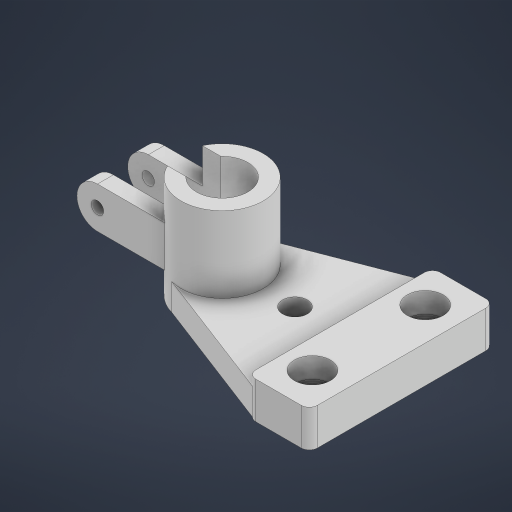
# Autodesk Inventor part: Part6
Saved by Autodesk Inventor 2023 (Build 270158000, 158)
## iProperties
Created: 2023-04-27
Part Number: Part6
Material: Ogólny
Document SubType Name: Modeling
Designer: Adam
Density: 1 g/cm^3
Appearance: Domyślna
Author: Adam
Autodesk Inventor part; units mm, degrees
ref_plane "YZ Plane" through (0, 0, 0) normal (1, 0, 0) x (0, 1, 0)
ref_plane "XZ Plane" through (0, 0, 0) normal (0, 1, 0) x (-1, 0, 0)
ref_plane "XY Plane" through (0, 0, 0) normal (0, 0, 1) x (1, 0, 0)
sketch "Szkic1" plane through (0, 0, 0) normal (0, 1, 0) x (-1, 0, 0)
  line L0 (-8, -90) -> (-52, -90)
  line L1 (-60, -82) -> (-60, 82)
  line L2 (-52, 90) -> (-8, 90)
  line L3 (0, 82) -> (0, -82)
  arc A0 (-8, -90) -> (0, -82) centre (-8, -82) ccw
  arc A1 (-60, -82) -> (-52, -90) centre (-52, -82) ccw
  arc A2 (0, 82) -> (-8, 90) centre (-8, 82) ccw
  arc A3 (-52, 90) -> (-60, 82) centre (-52, 82) ccw
  line L4 (-2.3431, -87.6569) -> (125.3697, -38.6325)
  line L5 (-2.3431, -87.6569) -> (134.4558, -87.6569) construction
  line L6 (-2.3431, 87.6569) -> (125.3697, 38.6325)
  line L7 (-2.3431, 87.6569) -> (134.4558, 87.6569) construction
  line L8 (193.533, -17) -> (224, -17)
  line L9 (224, 17) -> (193.533, 17)
  line L10 (193.533, -17) -> (133.3303, -17)
  line L11 (193.533, 17) -> (133.3303, 17)
  line L12 (224, -17) -> (224, -32.5)
  line L13 (224, 17) -> (224, 32.5)
  line L14 (224, 32.5) -> (138.3184, 32.5)
  line L15 (224, -32.5) -> (138.3184, -32.5)
  arc A4 (133.3303, 17) -> (133.3303, -17) centre (115, 0) ccw
  arc A5 (151.2077, 17) -> (151.2077, -17) centre (115, 0) ccw
  point P0 (0, 0)
  point P1 (-60, 90)
  point P2 (-60, -90)
  point P3 (0, 90)
  point P4 (-30, 0)
  point P5 (125.3697, 38.6325)
  dimension "d0" = 60
  dimension "d1" = 180
  dimension "d2" = 8
  dimension "d5" = 21
  dimension "d6" = 21
  dimension "d9" = 15.5
  dimension "d10" = 15.5
  constraints: 32 end point, 14 point on circle, 8 point on line, 8 tangent, 6 centre point, 5 horizontal, 5 parallel, 3 equal radius, 2 equal length, 2 perpendicular, 2 vertical, 1 midpoint
  measures "d0" distance of point (-60, 90) point (0, 90)
  measures "d1" distance of point (-60, -90) point (-60, 90)
  measures "d2" radius of A0
  measures "d5" angle of L5 L4
  measures "d6" angle of L6 L7
  measures "d9" distance of L8.end L12.end
  measures "d10" distance of L9.start L13.end
extrude "Wyciągnięcie proste1" add sketch "Szkic1" along normal blind 100
sketch "Szkic2" plane through (0, 100, 0) normal (0, 1, 0) x (1, 0, 0)
  line L0 (8, -90) -> (52, -90)
  line L1 (60, -82) -> (60, 82)
  line L2 (52, 90) -> (8, 90)
  line L3 (0, 82) -> (0, -82)
  arc A0 (0, -82) -> (8, -90) centre (8, -82) ccw
  arc A1 (8, 90) -> (0, 82) centre (8, 82) ccw
  arc A2 (60, 82) -> (52, 90) centre (52, 82) ccw
  arc A3 (52, -90) -> (60, -82) centre (52, -82) ccw
  point P0 (0, 0)
  dimension "d13" = 8
  constraints: 8 end point, 8 point on circle, 8 tangent, 4 centre point, 3 equal radius, 2 parallel, 1 horizontal, 1 perpendicular
  measures "d13" radius of A0
extrude "Wyciągnięcie proste2" cut sketch "Szkic2" against normal blind 64
sketch "Szkic3" plane through (0, 100, 0) normal (0, 1, 0) x (1, 0, 0)
  arc A0 (-138.3184, -32.5) -> (-125.3697, -38.6325) centre (-115, 0) ccw projected
  arc A1 (-125.3697, 38.6325) -> (-138.3184, 32.5) centre (-115, 0) ccw projected
  arc A2 (-138.3184, -32.5) -> (-138.3184, 32.5) centre (-115, 0) ccw
  line L0 (-125.3697, -38.6325) -> (2.3431, -87.6569) projected
  line L1 (-125.3697, -38.6325) -> (2.3431, -87.6569)
  line L2 (2.3431, 87.6569) -> (-125.3697, 38.6325) projected
  line L3 (-125.3697, 38.6325) -> (2.3431, 87.6569)
  line L4 (0, -82) -> (0, 82) projected
  line L5 (0, -82) -> (0, 82)
  arc A3 (0, -82) -> (2.3431, -87.6569) centre (8, -82) ccw projected
  arc A4 (0, -82) -> (2.3431, -87.6569) centre (8, -82) ccw
  arc A5 (8, 90) -> (2.3431, 87.6569) centre (8, 82) ccw projected
  arc A6 (8, 90) -> (0, 82) centre (8, 82) ccw
  point P0 (0, 0)
  point P1 (-125.3697, 38.6325)
  point P2 (-125.3697, -38.6325)
  constraints: 6 end point, 6 point on circle, 3 centre point, 3 collinear, 1 tangent
extrude "Wyciągnięcie proste3" cut sketch "Szkic3" against normal blind 74
sketch "Szkic4" plane through (0, 0, 0) normal (0, -1, 0) x (1, 0, 0)
  line L0 (-224, 32.5) -> (-138.3184, 32.5) projected
  line L1 (-224, 32.5) -> (-138.3184, 32.5)
  line L2 (-224, 17) -> (-224, 32.5) projected
  line L3 (-224, 32.5) -> (-224, 17)
  arc A0 (-125.3697, 38.6325) -> (-138.3184, 32.5) centre (-115, 0) ccw projected
  arc A1 (-138.3184, 32.5) -> (-151.2077, 17) centre (-115, 0) ccw
  line L4 (-133.3303, 17) -> (-224, 17) projected
  line L5 (-224, 17) -> (-151.2077, 17)
  arc A2 (-138.3184, -32.5) -> (-125.3697, -38.6325) centre (-115, 0) ccw projected
  arc A3 (-151.2077, -17) -> (-137.5648, -33.0277) centre (-115, 0) ccw
  line L6 (-224, -17) -> (-133.3303, -17) projected
  line L7 (-151.2077, -17) -> (-224, -17)
  line L8 (-224, -32.5) -> (-224, -17) projected
  line L9 (-224, -17) -> (-224, -32.5)
  line L10 (-224, -32.5) -> (-138.3184, -32.5)
  point P0 (0, 0)
  point P1 (-138.3184, -32.5)
  dimension "d18" = 40
  constraints: 12 end point, 5 collinear, 5 point on circle, 2 centre point, 1 perpendicular
  measures "d18" radius of A1
extrude "Wyciągnięcie proste4" cut sketch "Szkic4" against normal blind 26
sketch "Szkic5" plane through (0, 100, 0) normal (0, 1, 0) x (1, 0, 0)
  arc A0 (-138.3184, 32.5) -> (-151.2077, 17) centre (-115, 0) ccw projected
  arc A1 (-138.3184, 32.5) -> (-151.2077, 17) centre (-115, 0) ccw
  arc A2 (-151.2077, -17) -> (-125.3697, -38.6325) centre (-115, 0) ccw projected
  line L0 (-224, -32.5) -> (-138.3184, -32.5) projected
  arc A3 (-151.2077, -17) -> (-138.3184, -32.5) centre (-115, 0) ccw
  line L1 (-138.3184, 32.5) -> (-224, 32.5) projected
  line L2 (-138.3184, 32.5) -> (-224, 32.5)
  line L3 (-224, 32.5) -> (-224, 17) projected
  line L4 (-224, 32.5) -> (-224, 17)
  line L5 (-224, 17) -> (-151.2077, 17)
  line L6 (-133.3303, -17) -> (-224, -17) projected
  line L7 (-151.2077, -17) -> (-224, -17)
  line L8 (-224, -17) -> (-224, -32.5) projected
  line L9 (-224, -17) -> (-224, -32.5)
  line L10 (-224, -32.5) -> (-138.3184, -32.5)
  point P0 (0, 0)
  constraints: 12 end point, 5 point on circle, 3 collinear, 3 perpendicular, 2 centre point, 1 concentric
extrude "Wyciągnięcie proste5" cut sketch "Szkic5" against normal blind 34
sketch "Szkic6" plane through (-224, 26, 32.5) normal (0, 0, 1) x (1, 0, 0)
  point P0 (224, -26)
sketch "Szkic7" plane through (0, 36, 0) normal (0, 1, 0) x (1, 0, 0)
  line L0 (8, 90) -> (52, 90) projected
  line L1 (60, 82) -> (60, -82) projected
  point P0 (0, 0)
  point P1 (28, 55)
  point P2 (30, 90)
  point P3 (28, -55)
  dimension "d23" = 35
  dimension "d24" = 32
  constraints: 1 midpoint
  measures "d23" vertical distance of point (28, 55) point (30, 90)
  measures "d24" distance from line of L1 point (28, 55)
sketch "Szkic8" plane through (0, 26, 0) normal (0, 1, 0) x (1, 0, 0)
  point P0 (0, 0)
  point P1 (44, 0)
  point P2 (44, 0)
  point P3 (-44, 0)
  constraints: 1 coincident
hole "Otwór1" at (-44, 26, 0) direction (0, -1, 0) diameter 24 end through all
hole "Otwór2" at (28, 36, -55) at (28, 36, 55) direction (0, -1, 0) diameter 25 end through all counterbore diameter 35 counterbore depth 20
sketch "Szkic9" plane through (-224, 26, 32.5) normal (0, 0, 1) x (1, 0, 0)
  point P0 (224, -26)
sketch "Szkic10" plane through (-224, 26, 32.5) normal (0, 0, 1) x (1, 0, 0)
  point P0 (224, -26)
  point P1 (20, 20)
hole "Otwór3" at (-204, 46, 32.5) direction (0, 0, -1) diameter 12 end through all
full round fillet "Zaokrąglenie pełne1" first side at (-199.7359, 66, -22.1667) centre faces at (-224, 39.3333, -27.3333) second side at (-199.7359, 26, -22.1667)
full round fillet "Zaokrąglenie pełne2" first side at (-199.7359, 66, 22.1667) centre faces at (-224, 39.3333, 22.1667) second side at (-199.7359, 26, 22.1667)
